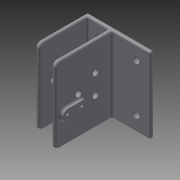
# Autodesk Inventor part: bed-stopper
Saved by Autodesk Inventor 2014 (Build 180170000, 170)
## iProperties
Created: 2017-07-21
Part Number: bed-stopper
Material: 一般
Document SubType Name: Modeling
Designer: hide
Density: 1 g/cm^3
Appearance: 既定
Author: hide
Autodesk Inventor part; units mm, degrees
ref_plane "YZ Plane" through (0, 0, 0) normal (1, 0, 0) x (0, 1, 0)
ref_plane "XZ Plane" through (0, 0, 0) normal (0, 1, 0) x (-1, 0, 0)
ref_plane "XY Plane" through (0, 0, 0) normal (0, 0, 1) x (1, 0, 0)
sketch "スケッチ1" plane through (0, 0, 0) normal (0, 0, 1) x (1, 0, 0)
  line L0 (0, -51) -> (0, 0)
  line L1 (22, 0) -> (22, -60)
  line L2 (22, -60) -> (26, -60)
  line L3 (26, -60) -> (26, 4)
  line L4 (26, 4) -> (-4, 4)
  line L5 (-4, 4) -> (-4, -51)
  line L6 (-4, -51) -> (0, -51)
  line L7 (0, 0) -> (22, 0)
  line L8 (26, 4) -> (66, 4)
  line L9 (66, 4) -> (66, 0)
  line L10 (66, 0) -> (26, 0)
  line L11 (26, 0) -> (26, 4)
  dimension "d0" = 4
  dimension "d1" = 4
  dimension "d2" = 4
  dimension "d3" = 60
  dimension "d4" = 22
  dimension "d5" = 55
  dimension "d81" = 4
  dimension "d82" = 40
  constraints: 24 end point, 8 parallel, 2 perpendicular, 1 horizontal, 1 vertical
  measures "d0" distance between parallel lines of L4 L7
  measures "d1" distance between parallel lines of L5 L0
  measures "d2" distance between parallel lines of L3 L1
  measures "d3" distance between parallel lines of L7 L2
  measures "d4" distance between parallel lines of L0 L1
  measures "d5" distance between parallel lines of L4 L6
  measures "d81" distance between parallel lines of L8 L10
  measures "d82" distance between parallel lines of L3 L9
extrude "押し出し1" add sketch "スケッチ1" along normal blind 80
sketch "スケッチ2" plane through (-4, -51, 0) normal (-1, 0, 0) x (0, 0, 1)
  line L0 (0, 0) -> (0, 55) projected
  line L1 (0, 55) -> (80, 55) projected
  line L2 (22.5, 45) -> (57.5, 45)
  line L3 (57.5, 45) -> (57.5, 10)
  line L4 (57.5, 10) -> (22.5, 10)
  line L5 (22.5, 10) -> (22.5, 45)
  point P0 (0, 51)
  dimension "d8" = 35
  dimension "d9" = 35
  dimension "d10" = 22.5
  dimension "d11" = 10
  constraints: 8 end point, 2 parallel, 1 horizontal, 1 perpendicular
  measures "d8" distance of L4.end L2.start
  measures "d9" distance of L2.start L2.end
  measures "d10" distance between parallel lines of L5 L0
  measures "d11" distance between parallel lines of L2 L1
extrude "押し出し2" add sketch "スケッチ2" along normal blind 5
fillet "フィレット1" radius 17.5 4 edges at (-6.5, -6, 22.5) (-6.5, -6, 57.5) (-6.5, -41, 22.5) (-6.5, -41, 57.5)
sketch "スケッチ3" plane through (-9, -51, 0) normal (-1, 0, 0) x (0, 0, 1)
  circle A0 centre (40, 15.5) radius 1.75
  circle A1 centre (40, 27.5) radius 17.5 projected
  circle A2 centre (50.3923, 33.5) radius 1.75
  circle A3 centre (29.6077, 33.5) radius 1.75
  point P0 (0, 51)
  dimension "d15" = 3.5
  dimension "d66" = 0
  dimension "d68" = 12
  dimension "d71" = 360
  constraints: 3 centre point, 7 other
  measures "d15" diameter of A0
  measures "d66" horizontal distance of A0.centre A1.centre
  measures "d68" distance of A1.centre A0.centre
extrude "押し出し3" cut sketch "スケッチ3" against normal blind 200 contours A0 | A2 | A3
fillet "フィレット2" radius 5 4 edges at (24, -60, 0) (24, -60, 80) (-2, -51, 0) (-2, -51, 80)
fillet "フィレット3" radius 1.8 32 edges at (22, 0, 40) (0, 0, 40) (-4, 4, 40) (-4, -49.5355, 78.5355) (-4, -21, 80) (-4, -49.5355, 1.4645) (-4, -21, 0) (-4, -51, 40) (26, -58.5355, 1.4645) (26, -60, 40) (26, -27.5, 0) (31, 4, 0) (0, -49.5355, 1.4645) (0, -51, 40) (0, -49.5355, 78.5355) (0, -23, 80) (0, -23, 0) (22, -58.5355, 1.4645) (22, -60, 40) (22, -27.5, 0) (11, 0, 0) (22, -58.5355, 78.5355) (22, -27.5, 80) (31, 4, 80) (11, 0, 80) (66, 4, 40) (46, 0, 0) (26, 0, 40) (66, 0, 40) (66, 2, 80) (66, 2, 0) (46, 0, 80)
sketch "スケッチ4" plane through (-9, -51, 0) normal (-1, 0, 0) x (0, 0, 1)
  circle A0 centre (40, 27.5) radius 17.5 projected
  line L0 (36, 47.9865) -> (44, 47.9865)
  line L1 (44, 47.9865) -> (44, 23.7409)
  line L2 (44, 23.7409) -> (36, 23.7409)
  line L3 (36, 23.7409) -> (36, 47.9865)
  point P0 (0, 51)
  dimension "d73" = 8
  dimension "d74" = 4
  constraints: 8 end point, 2 parallel, 1 horizontal, 1 perpendicular
  measures "d73" distance between parallel lines of L1 L3
  measures "d74" distance from line of A0.centre L1
extrude "押し出し4" cut sketch "スケッチ4" against normal blind 5 contours L1 L2 L3 A0 | A0 L3 L0 L1 picked at (39.552, 30.81)
sketch "スケッチ5" plane through (0, -46, 1.8) normal (1, 0, 0) x (0, 0, -1)
  circle A0 centre (-38.2, 10.5) radius 1.75 projected
  circle A1 centre (-38.2, 10.5) radius 3
  circle A2 centre (-27.8077, 28.5) radius 1.75 projected
  circle A3 centre (-48.5923, 28.5) radius 1.75 projected
  circle A4 centre (-48.5923, 28.5) radius 3
  circle A5 centre (-27.8077, 28.5) radius 3
  point P0 (1.8, 46)
  dimension "d28" = 6
  dimension "d75" = 6
  dimension "d76" = 6
  constraints: 3 centre point, 3 coincident
  measures "d28" diameter of A1
  measures "d75" diameter of A4
  measures "d76" diameter of A5
extrude "押し出し5" cut sketch "スケッチ5" along normal blind 100 and the other way blind 6.5
fillet "フィレット4" radius 5 7 edges at (-4, -35.8744, 27.6256) (-4, -23.5, 22.5) (-4, -12.6314, 26.2841) (-4, -12.6314, 53.7159) (-4, -23.5, 57.5) (-4, -35.8744, 52.3744) (-4, -41, 40)
sketch "スケッチ7" plane through (26, -55, 78.2) normal (1, 0, 0) x (0, 0, -1)
  circle A0 centre (38.2, 19.5) radius 3 projected
  line L0 (0, 0) -> (0, 53.2) projected
  arc A1 (0, 0) -> (3.2, -3.2) centre (3.2, 0) ccw projected
  line L1 (73.2, -3.2) -> (3.2, -3.2) projected
  arc A2 (73.2, -3.2) -> (76.4, 0) centre (73.2, 0) ccw projected
  line L2 (76.4, 53.2) -> (76.4, 0) projected
  circle A3 centre (48.2, 5) radius 3 projected
  circle A4 centre (48.2, 20) radius 3 projected
  circle A5 centre (48.2, 20) radius 1.25
  circle A6 centre (48.2, 5) radius 1.25
  line L3 (0, 53.2) -> (76.4, 53.2) projected
  point P0 (78.2, 55)
  dimension "d45" = 2.5
  dimension "d46" = 2.5
  constraints: 2 centre point, 2 coincident
  measures "d45" diameter of A5
  measures "d46" diameter of A6
extrude "押し出し7" cut sketch "スケッチ7" against normal blind 6 contours A5 | A6
sketch "スケッチ10" plane through (26, -55, 78.2) normal (1, 0, 0) x (0, 0, -1)
  circle A0 centre (48.2, 5) radius 1.25 projected
  circle A1 centre (48.2, 20) radius 1.25 projected
  line L0 (0, 0) -> (0, 53.2) projected
  line L1 (48.2, 20) -> (48.2, 5) construction
  line L2 (43.2, 20) -> (43.2, 5)
  line L3 (53.2, 5) -> (53.2, 20)
  arc A2 (53.2, 20) -> (43.2, 20) centre (48.2, 20) ccw
  arc A3 (43.2, 5) -> (53.2, 5) centre (48.2, 5) ccw
  point P0 (0, 57.2)
  point P1 (78.2, 55)
  point P2 (48.2, 12.5)
  point P3 (0, 55)
  dimension "d77" = 10
  constraints: 8 end point, 4 point on circle, 4 tangent, 2 centre point, 2 parallel, 1 midpoint
  measures "d77" distance between parallel lines of L3 L2
extrude "押し出し10" add sketch "スケッチ10" along normal blind 3
fillet "フィレット7" radius 3 4 edges at (26, -30, 30) (26, -42.5, 25) (26, -55, 30) (26, -42.5, 35)
sketch "スケッチ11" plane through (-2.2, 4, 78.2) normal (0, 1, 0) x (1, 0, 0)
  circle A0 centre (13.2, 62.3746) radius 5
  circle A1 centre (13.0562, 12.3748) radius 5
  circle A2 centre (53.2, 62.3746) radius 5
  circle A3 centre (53.2, 12.3746) radius 5
  line L0 (-1.8, 76.4) -> (-1.8, 0) projected
  point P0 (2.2, 78.2)
  dimension "d83" = 10
  dimension "d84" = 10
  dimension "d85" = 10
  dimension "d86" = 10
  dimension "d87" = 50
  dimension "d88" = 0
  dimension "d89" = 50
  dimension "d90" = 0
  dimension "d91" = 40
  dimension "d92" = 15
  constraints: 4 centre point
  measures "d83" diameter of A0
  measures "d84" diameter of A1
  measures "d85" diameter of A2
  measures "d86" diameter of A3
  measures "d87" distance of A1.centre A0.centre
  measures "d88" horizontal distance of A3.centre A2.centre
  measures "d89" distance of A3.centre A2.centre
  measures "d90" vertical distance of A2.centre A0.centre
  measures "d91" distance of A2.centre A0.centre
  measures "d92" distance from line of A0.centre L0
extrude "押し出し11" add sketch "スケッチ11" along normal blind 4
fillet "フィレット8" radius 4 4 edges at (6, 4, 15.8254) (46, 4, 15.8254) (46, 4, 65.8254) (5.8562, 4, 65.8252)
sketch "スケッチ12" plane through (10.8562, 8, 65.8252) normal (0, 1, 0) x (1, 0, 0)
  circle A0 centre (0, 0) radius 5 projected
  circle A1 centre (0.1438, 49.9998) radius 5 projected
  circle A2 centre (40.1438, 49.9998) radius 5 projected
  circle A3 centre (40.1438, -0.0002) radius 5 projected
  circle A4 centre (0.1438, 49.9998) radius 1.75
  circle A5 centre (40.1438, 49.9998) radius 1.75
  circle A6 centre (0, 0) radius 1.75
  circle A7 centre (40.1438, -0.0002) radius 1.75
  point P0 (-10.8562, 65.8252)
  dimension "d96" = 3.5
  dimension "d97" = 3.5
  dimension "d98" = 3.5
  dimension "d99" = 3.5
  constraints: 4 centre point, 4 coincident
  measures "d96" diameter of A4
  measures "d97" diameter of A5
  measures "d98" diameter of A6
  measures "d99" diameter of A7
extrude "押し出し12" cut sketch "スケッチ12" against normal blind 40 contours A4 | A5 | A6 | A7
sketch "スケッチ13" plane through (1.8, 0, 78.2) normal (0, -1, 0) x (1, 0, 0)
  circle A0 centre (9.0562, -12.3748) radius 1.75 projected
  circle A1 centre (9.2, -62.3746) radius 1.75 projected
  circle A2 centre (9.0562, -12.3748) radius 3.5
  circle A3 centre (49.2, -62.3746) radius 1.75 projected
  circle A4 centre (49.2, -12.3746) radius 1.75 projected
  line L0 (62.4, -76.4) -> (26, -76.4) projected
  line L1 (62.4, 0) -> (62.4, -76.4) projected
  line L2 (26, 0) -> (62.4, 0) projected
  line L3 (26, -76.4) -> (26, 0) projected
  circle A5 centre (49.2, -12.3746) radius 3.5
  circle A6 centre (9.2, -62.3746) radius 3.5
  circle A7 centre (49.2, -62.3746) radius 3.5
  point P0 (-1.8, -78.2)
  dimension "d102" = 7
  dimension "d103" = 7
  dimension "d104" = 7
  dimension "d105" = 7
  constraints: 4 centre point, 4 coincident
  measures "d102" diameter of A2
  measures "d103" diameter of A5
  measures "d104" diameter of A6
  measures "d105" diameter of A7
extrude "押し出し13" cut sketch "スケッチ13" against normal blind 4 contours A2 | A5 | A6 | A7
fillet "フィレット9" radius 1 4 edges at (7.3562, 4, 65.8252) (7.5, 4, 15.8254) (47.5, 4, 15.8254) (47.5, 4, 65.8254)
fillet "フィレット10" radius 3 3 edges at (-4, -14.3087, 36) (-4, -14.3087, 44) (-4, -27.2591, 40)
equation "\"d0\" = d2"
equation "\"d1\" = d2"
equation "\"d8\" = d9"
equation "\"d74\" = 0.5 * d73"
equation "\"d75\" = d28"
equation "\"d76\" = d28"
equation "\"d46\" = d45"
equation "\"d84\" = d83"
equation "\"d85\" = d84"
equation "\"d86\" = d84"
equation "\"d89\" = d87"
equation "\"d97\" = d96"
equation "\"d98\" = d96"
equation "\"d99\" = d96"
equation "\"d103\" = d102"
equation "\"d104\" = d102"
equation "\"d105\" = d102"
